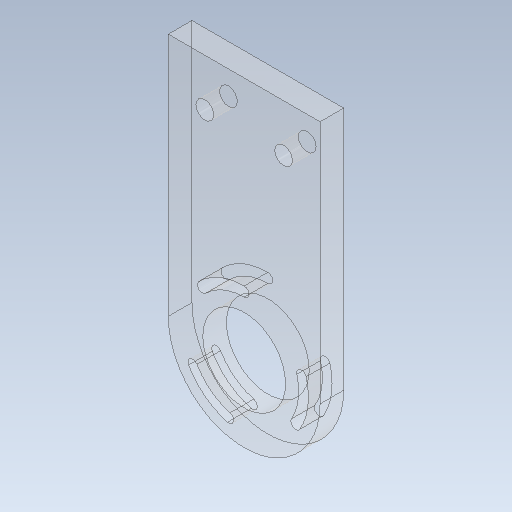
# Autodesk Inventor part: Joint1C_1
Saved by Autodesk Inventor 2021.1 (Build 251245010, 245A)
## iProperties
Created: 2023-10-21
Part Number: Joint1C_1
Material: PMMA Plastic
Document SubType Name: Modeling
Designer: user
Density: 1.188 g/cm^3
Appearance: Polycarbonate - Clear
Author: user
Autodesk Inventor part; units mm, degrees
ref_plane "YZ Plane" through (0, 0, 0) normal (1, 0, 0) x (0, 1, 0)
ref_plane "XZ Plane" through (0, 0, 0) normal (0, 1, 0) x (-1, 0, 0)
ref_plane "XY Plane" through (0, 0, 0) normal (0, 0, 1) x (1, 0, 0)
sketch "Sketch1" plane through (0, 0, 0) normal (0, 0, 1) x (1, 0, 0)
  arc A0 (-19.25, -19.25) -> (19.25, -19.25) centre (0, -19.25) ccw
  circle A1 centre (0, -19.25) radius 10.5
  arc A2 (11.9852, -26.1697) -> (14.1148, -27.3992) centre (13.05, -26.7844) ccw
  arc A3 (-11.9852, -26.1697) -> (-14.1148, -27.3992) centre (-13.05, -26.7844) ccw
  arc A4 (0, -5.4107) -> (0, -2.9517) centre (0, -4.1812) ccw
  line L0 (0, -19.25) -> (14.5554, -15.3499) construction
  line L1 (0, -19.25) -> (13.05, -26.7844) construction
  line L2 (0, -19.25) -> (-10.6553, -8.5947) construction
  line L3 (0, -19.25) -> (0, -4.1812) construction
  line L4 (0, -19.25) -> (-3.9001, -33.8054) construction
  line L5 (0, -19.25) -> (-13.05, -26.7844) construction
  arc A5 (-4.2183, -34.993) -> (-3.5819, -32.6178) centre (-3.9001, -33.8054) ccw
  arc A6 (15.743, -15.0317) -> (13.3678, -15.6681) centre (14.5554, -15.3499) ccw
  arc A7 (-11.5247, -7.7253) -> (-9.7859, -9.4641) centre (-10.6553, -8.5947) ccw
  arc A8 (0, -2.9517) -> (-11.5247, -7.7253) centre (0, -19.25) ccw
  arc A9 (0, -5.4107) -> (-9.7859, -9.4641) centre (0, -19.25) ccw
  arc A10 (11.9852, -26.1697) -> (13.3678, -15.6681) centre (0, -19.25) ccw
  arc A11 (14.1148, -27.3992) -> (15.743, -15.0317) centre (0, -19.25) ccw
  arc A12 (-11.9852, -26.1697) -> (-3.5819, -32.6178) centre (0, -19.25) ccw
  arc A13 (-14.1148, -27.3992) -> (-4.2183, -34.993) centre (0, -19.25) ccw
  line L6 (19.25, -19.25) -> (19.25, 42.75)
  line L7 (-19.25, -19.25) -> (-19.25, 42.75)
  line L8 (19.25, 42.75) -> (-19.25, 42.75)
  circle A14 centre (-10, 30.75) radius 2.25
  circle A15 centre (10, 30.75) radius 2.25
  line L9 (10, 30.75) -> (-10, 30.75)
  point P0 (0, 0)
  point P1 (19.25, 30.75)
  dimension "d0" = 21
  dimension "d1" = 45
  dimension "d2" = 45
  dimension "d3" = 45
  dimension "d4" = 2.459
  dimension "d5" = 2.459
  dimension "d6" = 2.459
  dimension "d7" = 2.459
  dimension "d8" = 2.459
  dimension "d9" = 2.459
  dimension "d11" = 62
  dimension "d14" = 19.25
  dimension "d21" = 4.5
  dimension "d22" = 12
  dimension "d23" = 4.5
  dimension "d24" = 20
  dimension "d25" = 9.25
  dimension "d26" = 38.5
  constraints: 26 point on circle, 20 end point, 16 centre point, 13 coincident, 8 point on line, 2 horizontal, 2 tangent, 2 vertical, 5 other
  measures "d0" diameter of A1
  measures "d1" angle of L1 L0
  measures "d2" angle of L3 L2
  measures "d3" angle of L5 L4
  measures "d4" diameter of A3
  measures "d5" diameter of A5
  measures "d6" diameter of A6
  measures "d7" diameter of A7
  measures "d8" diameter of A2
  measures "d9" diameter of A4
  measures "d11" distance of L7.start L7.end
  measures "d14" radius of A0
  measures "d21" diameter of A14
  measures "d22" distance from line of L8 A14.centre
  measures "d23" diameter of A15
  measures "d24" distance of L9.start L9.end
  measures "d25" distance from line of L7 L9.end
  measures "d26" distance of L6.end L7.end
extrude "Extrusion1" add sketch "Sketch1" along normal blind 6
equation "\"d8\" = d6"
equation "\"d9\" = d7"
equation "\"d23\" = d21"
equation "\"d25\" = -0.5 * d24 + 0.5 * d26"
body "Solid1"
